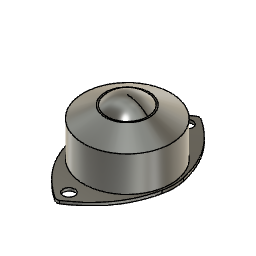
Roue Pivot v1 (Autodesk Fusion 360 design; units mm, degrees)
Autodesk Fusion 360 part; units mm, degrees
sketch "Esquisse1" plane through (0, 0, 0) normal (0, 0, 1) x (1, 0, 0)
  circle A0 centre (0, 0) radius 16
  line L0 (0, 25) -> (0, -25)
  line L1 (0, 16) -> (0, 25)
  circle A1 centre (0, 20.5) radius 2
  spline S0 degree 5 poles (-15.998, 0.25) (-15.7389, 1.9932) (-15.1133, 5.2622) (-13.8531, 9.5141) (-11.6152, 14.0579) (-8.1767, 18.4749) (-5.0788, 21.3679) (-2.5998, 23.2801) (-0.8781, 24.445) (0, 25) knots 0 0 0 0 0 0 0.2 0.4 0.6 0.8 1 1 1 1 1 1
  line L2 (-16.6171, -3.9145) -> (-15.379, 4.4145)
  spline S1 degree 5 poles (15.998, 0.25) (15.7389, 1.9932) (15.1133, 5.2622) (13.8531, 9.5141) (11.6152, 14.0579) (8.1767, 18.4749) (5.0788, 21.3679) (2.5998, 23.2801) (0.8781, 24.445) (0, 25) knots 0 0 0 0 0 0 0.2 0.4 0.6 0.8 1 1 1 1 1 1
  line L3 (-2.0948, 23.676) -> (2.0948, 26.324)
  line L4 (16.6171, -3.9145) -> (15.379, 4.4145)
  line L5 (2.0948, 23.676) -> (-2.0948, 26.324)
  line L6 (-15.998, 0.25) -> (15.998, 0.25)
  spline S2 degree 5 poles (-15.998, 0.25) (-15.7389, -1.4932) (-15.1133, -4.7622) (-13.8531, -9.0141) (-11.6152, -13.5579) (-8.1767, -17.9749) (-5.0788, -20.8679) (-2.5998, -22.7801) (-0.8781, -23.945) (0, -24.5) knots 0 0 0 0 0 0 0.2 0.4 0.6 0.8 1 1 1 1 1 1
  line L7 (-16.6171, 4.4145) -> (-15.379, -3.9145)
  line L8 (-2.0948, -23.176) -> (2.0948, -25.824)
  spline S3 degree 5 poles (15.998, 0.25) (15.7389, -1.4932) (15.1133, -4.7622) (13.8531, -9.0141) (11.6152, -13.5579) (8.1767, -17.9749) (5.0788, -20.8679) (2.5998, -22.7801) (0.8781, -23.945) (0, -24.5) knots 0 0 0 0 0 0 0.2 0.4 0.6 0.8 1 1 1 1 1 1
  line L9 (16.6171, 4.4145) -> (15.379, -3.9145)
  line L10 (2.0948, -23.176) -> (-2.0948, -25.824)
  circle A2 centre (0, -20) radius 2
  point P0 (0, 16)
  dimension "d1" = 32
  dimension "d2" = 50
  dimension "d3" = 25
  dimension "d4" = 4
  constraint coincident A0.centre origin
  constraint vertical L0
  constraint coincident A0 P0
  constraint coincident L0 P0
  constraint midpoint L1 A1.centre
  constraint coincident A0 S0.start
  constraint midpoint S0.start L2
  constraint coincident A0 L2.end
  constraint midpoint L0.start L3
  constraint symmetric L1.end L0 S0.end
  constraint symmetric L0 P0 L1.start
  constraint symmetric L0 S0.start S1.start
  constraint symmetric L0 L2.start L4.start
  constraint symmetric L0 L2.end L4.end
  constraint symmetric L0 L3.start L5.start
  constraint symmetric L0 L3.end L5.end
  constraint symmetric L0.start L6 S2.end
  constraint symmetric A1 L6 A2
  constraint symmetric S0.start L6 S2.start
  constraint symmetric L2.start L6 L7.start
  constraint symmetric L2.end L6 L7.end
  constraint symmetric S1.start L6 S3.start
  constraint symmetric L3.start L6 L8.start
  constraint symmetric L3.end L6 L8.end
  constraint symmetric L4.start L6 L9.start
  constraint symmetric L4.end L6 L9.end
  constraint symmetric L5.start L6 L10.start
  constraint symmetric L5.end L6 L10.end
  measures "d1" diameter of A0
  measures "d2" distance of L0.start L0.end
  measures "d3" distance of A0.centre L0.start
  measures "d4" diameter of A1
extrude "Extrusion1" add sketch "Esquisse1" along normal blind 1 contours A0 L0 S1 L6 | A0 L0 L6 S3 | A0 L0 S3 A2 | A0 L0 L1 A1 S1 | A0 L0 S0 L6 | A0 L0 L6 S2 | A0 L0 S2 A2 | A0 L0 L1 A1 S0
sketch "Esquisse2" plane through (0, 0, 1) normal (0, 0, 1) x (-1, 0, 0)
  circle A0 centre (0, -20.5) radius 2
  circle A1 centre (0, 20) radius 2
  spline S0 degree 5 poles (15.998, -0.25) (15.7389, 1.4932) (15.1133, 4.7622) (13.8531, 9.0141) (11.6152, 13.5579) (8.1767, 17.9749) (5.0788, 20.8679) (2.5998, 22.7801) (0.8781, 23.945) (0, 24.5) knots 0 0 0 0 0 0 0.2 0.4 0.6 0.8 1 1 1 1 1 1
  spline S1 degree 5 poles (0, 24.5) (-0.8781, 23.945) (-2.5998, 22.7801) (-5.0788, 20.8679) (-8.1767, 17.9749) (-11.6152, 13.5579) (-13.8531, 9.0141) (-15.1133, 4.7622) (-15.7389, 1.4932) (-15.998, -0.25) knots -1 -1 -1 -1 -1 -1 -0.8 -0.6 -0.4 -0.2 0 0 0 0 0 0
  spline S2 degree 5 poles (-15.998, -0.25) (-15.7389, -1.9932) (-15.1133, -5.2622) (-13.8531, -9.5141) (-11.6152, -14.0579) (-8.1767, -18.4749) (-5.0788, -21.3679) (-2.5998, -23.2801) (-0.8781, -24.445) (0, -25) knots 0 0 0 0 0 0 0.2 0.4 0.6 0.8 1 1 1 1 1 1
  spline S3 degree 5 poles (0, -25) (0.8781, -24.445) (2.5998, -23.2801) (5.0788, -21.3679) (8.1767, -18.4749) (11.6152, -14.0579) (13.8531, -9.5141) (15.1133, -5.2622) (15.7389, -1.9932) (15.998, -0.25) knots -1 -1 -1 -1 -1 -1 -0.8 -0.6 -0.4 -0.2 0 0 0 0 0 0
  circle A2 centre (0, 0) radius 15
  dimension "d7" = 30
  constraint coincident A2.centre origin
  measures "d7" diameter of A2
extrude "Extrusion2" add sketch "Esquisse2" along normal blind 12 contours A2
fillet "Congé1" radius 1.5 2 edges at (0, -24.5, 0.5) (0, 25, 0.5)
sketch "Esquisse4" plane through (0, 0, 0) normal (0, 1, 0) x (1, 0, 0)
  line L0 (0, -13) -> (0, -17)
  line L1 (0, -17) -> (7.5, -17)
  line L2 (7.5, -17) -> (15, -13)
  line L3 (0, -13) -> (15, -13)
  dimension "d15" = 4
  dimension "d16" = 7.5
  constraint vertical L0
  constraint perpendicular L0 L1
  constraint perpendicular L0 L3
  measures "d15" distance of L0.start L0.end
  measures "d16" distance of L0.end L1.end
revolve "Révolution1" add sketch "Esquisse4" angle 360 about axis through (0, 0, 13) along (0, 0, 1)
sketch "Esquisse5" plane through (0, 0, 0) normal (0, 1, 0) x (1, 0, 0)
  line L0 (0, -17) -> (0, -20)
  spline S0 degree 5 poles (0, -20) (0.408, -20) (1.1867, -19.965) (2.2427, -19.8075) (3.4576, -19.4165) (4.7621, -18.7269) (5.7006, -18.0768) (6.3647, -17.5519) (6.791, -17.1866) (7, -17) knots 0 0 0 0 0 0 0.2 0.4 0.6 0.8 1 1 1 1 1 1
  line L1 (-1, -20) -> (1, -20)
  line L2 (0, -17) -> (7, -17)
  dimension "d18" = 20
  dimension "d19" = 7
  constraint vertical L0
  constraint midpoint L0.end L1
  constraint perpendicular L0 L2
  measures "d18" distance of origin L0.end
  measures "d19" distance of L0 S0.end
revolve "Révolution2" add sketch "Esquisse5" angle 360 about axis through (0, 0, 17) along (0, 0, 1)
fillet "Congé2" radius 16.5 2 edges at (15.998, 0.25, 0.5) (-15.998, 0.25, 0.5)
